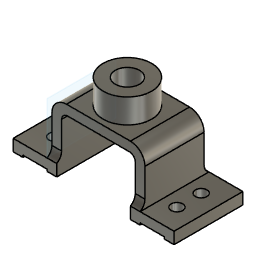
ORTHOGRAPHIC PROJECTIONS_SHEET_DRAWING_1 (Autodesk Fusion 360 design; units mm, degrees)
Autodesk Fusion 360 part; units mm, degrees
sketch "Sketch1" plane through (0, 0, 0) normal (0, 1, 0) x (1, 0, 0)
  line L0 (0, 0) -> (83, 0)
  line L1 (-83, 0) -> (-83, 6)
  line L2 (-83, 0) -> (-83, -6)
  line L3 (-83, 6) -> (-73, 6)
  line L4 (-73, 6) -> (-73, 4)
  line L5 (-73, 4) -> (-48, 4)
  line L6 (-48, 4) -> (-48, 6)
  line L7 (-48, 6) -> (-38, 6)
  line L8 (-83, -6) -> (-48, -6)
  line L9 (-38, -6) -> (-38, 6)
  line L10 (-38, -6) -> (-38, -49)
  line L11 (-48, -49) -> (-48, -6)
  line L12 (-38, -49) -> (0, -49)
  line L13 (0, -49) -> (0, -59)
  line L14 (0, -59) -> (-48, -59)
  line L15 (-48, -59) -> (-48, -49)
  dimension "d1" = 83
  dimension "d2" = 83
  dimension "d3" = 6
  dimension "d4" = 6
  dimension "d5" = 10
  dimension "d6" = 2
  dimension "d7" = 25
  dimension "d8" = 2
  dimension "d9" = 10
  dimension "d10" = 43
  dimension "d11" = 10
  dimension "d12" = 10
  constraint coincident L0.start origin
  constraint perpendicular L1 L3
  constraint perpendicular L3 L4
  constraint perpendicular L4 L5
  constraint perpendicular L5 L6
  constraint perpendicular L6 L7
  constraint perpendicular L2 L8
  constraint perpendicular L7 L9
  constraint perpendicular L8 L10
  constraint perpendicular L8 L11
  constraint perpendicular L10 L12
  constraint perpendicular L12 L13
  constraint perpendicular L11 L14
  measures "d1" distance of L0.start L1.start
  measures "d2" distance of L0.start L0.end
  measures "d3" distance of L1.start L1.end
  measures "d4" distance of L1.start L2.end
  measures "d5" distance of L1.end L3.end
  measures "d6" distance of L3.end L4.end
  measures "d7" distance of L4.end L5.end
  measures "d8" distance of L5.end L6.end
  measures "d9" distance of L6.end L7.end
  measures "d10" distance of L9.start L10.end
  measures "d11" distance of L10.end L11.start
  measures "d12" distance of L12.end L13.end
sketch "Sketch2" plane through (0, 0, 0) normal (0, 1, 0) x (1, 0, 0)
  line L0 (0, -65) -> (0, 0)
  line L1 (0, -49) -> (-38, -49)
  line L2 (-38, -49) -> (-38, 6)
  line L3 (-38, 6) -> (-48, 6)
  line L4 (-48, 6) -> (-48, 4)
  line L5 (-48, 4) -> (-73, 4)
  line L6 (-73, 4) -> (-73, 6)
  line L7 (-73, 6) -> (-83, 6)
  line L8 (-83, 6) -> (-83, -6)
  line L9 (-83, -6) -> (-49, -6)
  line L10 (-49, -6) -> (-48, -6)
  line L11 (-48, -6) -> (-48, -59)
  line L12 (-48, -59) -> (0, -59)
  line L13 (49, -6) -> (48, -6)
  line L14 (48, -6) -> (48, -59)
  line L15 (38, 6) -> (48, 6)
  line L16 (48, -59) -> (0, -59)
  line L17 (73, 4) -> (73, 6)
  line L18 (38, -49) -> (38, 6)
  line L19 (48, 4) -> (73, 4)
  line L20 (83, 6) -> (83, -6)
  line L21 (0, -65) -> (0, 0)
  line L22 (83, -6) -> (49, -6)
  line L23 (48, 6) -> (48, 4)
  line L24 (0, -49) -> (38, -49)
  line L25 (73, 6) -> (83, 6)
  constraint coincident L0.end L21.end
  constraint vertical L0
  constraint symmetric L21.end L0 origin
  constraint coincident L0 L1.start
  constraint perpendicular L0 L1
  constraint perpendicular L1 L2
  constraint perpendicular L0 L3
  constraint perpendicular L3 L4
  constraint perpendicular L4 L5
  constraint perpendicular L3 L6
  constraint perpendicular L6 L7
  constraint perpendicular L7 L8
  constraint perpendicular L8 L9
  constraint perpendicular L8 L10
  constraint perpendicular L10 L11
  constraint coincident L0 L12.end
  constraint perpendicular L0 L12
  constraint symmetric L21.start L0 L0.start
  constraint symmetric L0 L21.end origin
  constraint symmetric L0 L1.start L24.start
  constraint symmetric L0 L1.end L18.start
  constraint symmetric L0 L2.end L15.start
  constraint symmetric L0 L3.end L15.end
  constraint symmetric L0 L4.end L19.start
  constraint symmetric L0 L5.end L17.start
  constraint symmetric L0 L6.end L17.end
  constraint symmetric L0 L7.end L20.start
  constraint symmetric L0 L8.end L20.end
  constraint symmetric L0 L9.end L13.start
  constraint symmetric L0 L10.end L13.end
  constraint symmetric L0 L11.end L14.end
  constraint symmetric L0 L12.end L16.end
extrude "Extrude1" add sketch "Sketch1" sketch "Sketch2" along normal blind 71 of sketch 2 contours L0 L13 L14 L15 L16 L17 L18 L19 L20 L21 L22 L23 L24 L25
sketch "Sketch3" plane through (0, 0, 59) normal (0, 0, 1) x (-1, 0, 0)
  line L0 (48, 0) -> (-48, 0)
  line L1 (-48, 0) -> (-48, -71)
  line L2 (-48, -71) -> (48, -71)
  line L3 (48, -71) -> (48, 0)
  circle A0 centre (0.6463, -35.5) radius 25
  dimension "d16" = 50
  measures "d16" diameter of A0
extrude "Extrude2" add sketch "Sketch3" along normal blind 25 contours A0
sketch "Sketch4" plane through (0, 0, 84) normal (0, 0, 1) x (-1, 0, 0)
  circle A0 centre (0.6463, -35.5) radius 25
  circle A1 centre (0.6463, -35.5) radius 12.5
  dimension "d19" = 25
  constraint concentric A0 A1
  measures "d19" diameter of A1
extrude "Extrude3" cut sketch "Sketch4" against normal blind 25 contours A1
sketch "Sketch5" plane through (0, 0, 6) normal (0, 0, 1) x (-1, 0, 0)
  line L0 (-48, 0) -> (-83, 0)
  line L1 (-83, 0) -> (-83, -71)
  line L2 (-83, -71) -> (-48, -71)
  line L3 (-48, -71) -> (-48, 0)
  circle A0 centre (-63, -23) radius 6
  circle A1 centre (-63, -48) radius 6
  dimension "d25" = 12
  dimension "d28" = 12
  measures "d25" diameter of A0
  measures "d28" diameter of A1
sketch "Sketch6" plane through (-48, 0, 0) normal (-1, 0, 0) x (0, -1, 0)
  line L0 (0, 6) -> (0, 59)
  line L1 (0, 59) -> (-71, 59)
  line L2 (-71, 59) -> (-71, 6)
  line L3 (-71, 6) -> (0, 6)
sketch "Sketch7" plane through (0, 0, 6) normal (0, 0, 1) x (-1, 0, 0)
  line L0 (83, 0) -> (48, 0)
  line L1 (48, 0) -> (48, -71)
  line L2 (48, -71) -> (83, -71)
  line L3 (83, -71) -> (83, 0)
  line L4 (83, -48) -> (83, -23)
  circle A0 centre (63, -48) radius 6
  circle A1 centre (63, -23) radius 6
  line L5 (83, -23) -> (83, -48)
  dimension "d32" = 12
  dimension "d33" = 12
  measures "d32" diameter of A0
  measures "d33" diameter of A1
extrude "Extrude4" cut sketch "Sketch5" sketch "Sketch7" against normal blind 10 contours A0 | A1 of sketch 2 contours A0 | A1
sketch "Sketch8" plane through (-48, 0, 0) normal (-1, 0, 0) x (0, -1, 0)
sketch "Sketch9" plane through (0, 71, 0) normal (0, 1, 0) x (-1, 0, 0)
  line L0 (38, 49) -> (38, -6)
  line L1 (38, -6) -> (48, -6)
  line L2 (48, -6) -> (48, -4)
  line L3 (48, -4) -> (73, -4)
  line L4 (73, -4) -> (73, -6)
  line L5 (73, -6) -> (83, -6)
  line L6 (83, -6) -> (83, 6)
  line L7 (83, 6) -> (48, 6)
  line L8 (48, 6) -> (48, 59)
  line L9 (48, 59) -> (-48, 59)
  line L10 (-48, 59) -> (-48, 6)
  line L11 (-48, 6) -> (-83, 6)
  line L12 (-83, 6) -> (-83, -6)
  line L13 (-83, -6) -> (-73, -6)
  line L14 (-73, -6) -> (-73, -4)
  line L15 (-73, -4) -> (-48, -4)
  line L16 (-48, -4) -> (-48, -6)
  line L17 (-48, -6) -> (-38, -6)
  line L18 (-38, -6) -> (-38, 49)
  line L19 (-38, 49) -> (38, 49)
  line L20 (48, 6) -> (38, 6)
  line L21 (48, 6) -> (38, 6)
  line L22 (-48, 6) -> (-38, 6)
  line L23 (48, 6) -> (38, 6)
  constraint coincident L7.end L8.start
  constraint coincident L0 L20.end
  constraint perpendicular L0 L20
  constraint coincident L10.end L11.start
  constraint coincident L18 L22.end
  constraint perpendicular L18 L22
extrude "Extrude5" cut sketch "Sketch9" against normal blind 5 contours L0 L8 L9 L10 L18 L19 L20 L21 L22 L23
sketch "Sketch10" plane through (0, 0, 0) normal (0, -1, 0) x (1, 0, 0)
  line L0 (-38, -6) -> (-38, 49)
  line L1 (-38, 49) -> (38, 49)
  line L2 (38, 49) -> (38, -6)
  line L3 (38, -6) -> (48, -6)
  line L4 (48, -6) -> (48, -4)
  line L5 (48, -4) -> (73, -4)
  line L6 (73, -4) -> (73, -6)
  line L7 (73, -6) -> (83, -6)
  line L8 (83, -6) -> (83, 6)
  line L9 (83, 6) -> (48, 6)
  line L10 (48, 6) -> (48, 59)
  line L11 (48, 59) -> (-48, 59)
  line L12 (-48, 59) -> (-48, 6)
  line L13 (-48, 6) -> (-83, 6)
  line L14 (-83, 6) -> (-83, -6)
  line L15 (-83, -6) -> (-73, -6)
  line L16 (-73, -6) -> (-73, -4)
  line L17 (-73, -4) -> (-48, -4)
  line L18 (-48, -4) -> (-48, -6)
  line L19 (-48, -6) -> (-38, -6)
  line L20 (-48, 6) -> (-38, 6)
  line L21 (48, 6) -> (38, 6)
  constraint coincident L12.end L13.start
  constraint coincident L0 L20.end
  constraint perpendicular L0 L20
  constraint coincident L9.end L10.start
  constraint coincident L2 L21.end
  constraint perpendicular L2 L21
extrude "Extrude6" cut sketch "Sketch10" against normal blind 5 contours L0 L1 L2 L10 L11 L12 L20 L21
fillet "Fillet1" radius 10 1 edges at (-43, 66, 6)
fillet "Fillet2" radius 10 1 edges at (-43, 5, 6)
fillet "Fillet3" radius 10 1 edges at (43, 5, 6)
fillet "Fillet4" radius 10 1 edges at (43, 66, 6)
fillet "Fillet5" radius 15 1 edges at (-48, 35.5, 59)
fillet "Fillet6" radius 15 1 edges at (48, 35.5, 59)
fillet "Fillet7" radius 6 1 edges at (38, 35.5, 49)
fillet "Fillet8" radius 6 1 edges at (-38, 35.5, 49)
